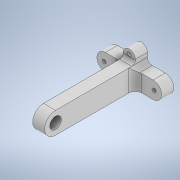
# Autodesk Inventor part: Motor Mount V2
Saved by Autodesk Inventor 2020 (Build 240168000, 168)
## iProperties
Created: 2022-04-04
Part Number: Motor Mount V2
Material: Generic
Document SubType Name: Modeling
Designer: maxwe
Density: 1 g/cm^3
Appearance: Default
Author: maxwe
Autodesk Inventor part; units mm, degrees
ref_plane "YZ Plane" through (0, 0, 0) normal (1, 0, 0) x (0, 1, 0)
ref_plane "XZ Plane" through (0, 0, 0) normal (0, 1, 0) x (-1, 0, 0)
ref_plane "XY Plane" through (0, 0, 0) normal (0, 0, 1) x (1, 0, 0)
sketch "Sketch1" plane through (0, 0, 0) normal (1, 0, 0) x (0, 1, 0)
  line L0 (0, 0) -> (17.9, 0)
  line L1 (17.9, 0) -> (17.9, 85)
  line L2 (17.9, 85) -> (0, 85)
  line L3 (0, 85) -> (0, 0)
  dimension "d0" = 17.9
  dimension "d1" = 85
  constraints: 8 end point, 2 parallel, 1 horizontal, 1 perpendicular
  measures "d0" distance of L2.end L1.end
  measures "d1" distance of L1.end L0.end
extrude "Extrusion1" add sketch "Sketch1" along normal blind 10
fillet "Fillet1" radius 8.95 2 edges at (5, 17.9, 85) (5, 0, 85)
sketch "Sketch2" plane through (10, 0, 0) normal (1, 0, 0) x (0, 0, -1)
  arc A0 (-76.05, 17.9) -> (-76.05, 0) centre (-76.05, 8.95) ccw projected
  circle A1 centre (-76.05, 8.95) radius 4.75
  point P0 (0, 0)
  dimension "d5" = 9.5
  constraints: 1 centre point, 1 coincident
  measures "d5" diameter of A1
extrude "Extrusion2" cut sketch "Sketch2" against normal blind 10
sketch "Sketch3" plane through (0, 0, 0) normal (0, 0, -1) x (-1, 0, 0)
  line L0 (14.8, 0) -> (-24.8, 0)
  line L1 (-31.8, 7) -> (-31.8, 7)
  line L2 (-24.8, 14) -> (14.8, 14)
  line L3 (21.8, 7) -> (21.8, 7)
  line L4 (0, 0) -> (0, 17.9) projected
  line L5 (-10, 0) -> (-10, 17.9) projected
  line L6 (0, 17.9) -> (-10, 17.9) projected
  circle A0 centre (-25.7, 7) radius 1.6
  circle A1 centre (15.7, 7) radius 1.6
  arc A2 (-24.8, 14) -> (-31.8, 7) centre (-24.8, 7) ccw
  arc A3 (-31.8, 7) -> (-24.8, 0) centre (-24.8, 7) ccw
  arc A4 (21.8, 7) -> (14.8, 14) centre (14.8, 7) ccw
  arc A5 (14.8, 0) -> (21.8, 7) centre (14.8, 7) ccw
  point P0 (21.8, 0)
  point P1 (-31.8, 14)
  point P2 (-31.8, 0)
  point P3 (21.8, 14)
  point P4 (-10, 14)
  point P5 (0, 14)
  point P6 (21.8, 7)
  point P7 (-31.8, 7)
  dimension "d8" = 14
  dimension "d9" = 21.8
  dimension "d10" = 21.8
  dimension "d11" = 17.9
  dimension "d12" = 3.2
  dimension "d13" = 3.2
  dimension "d14" = 6.1
  dimension "d15" = 6.1
  dimension "d16" = 7
  dimension "d17" = 7
  dimension "d23" = 7
  constraints: 8 end point, 8 point on circle, 8 point on line, 8 tangent, 6 centre point, 3 equal radius, 2 parallel, 1 horizontal, 1 perpendicular
  measures "d8" distance of point (21.8, 14) point (21.8, 0)
  measures "d9" distance between parallel lines of L4 L3
  measures "d10" distance between parallel lines of L5 L1
  measures "d11" distance between parallel lines of L6 L0
  measures "d12" diameter of A0
  measures "d13" diameter of A1
  measures "d14" distance from line of L1 A0.centre
  measures "d15" distance from line of L3 A1.centre
  measures "d16" distance from line of L2 A0.centre
  measures "d17" distance from line of L2 A1.centre
  measures "d23" radius of A2
extrude "Extrusion3" add sketch "Sketch3" against normal blind 10 contours L0 L4 L2 A4 A5 | L0 L5 L2 L4 | L0 A3 A2 L2 L5
fillet "Fillet3" radius 5.5 2 edges at (10, 7, 10) (0, 7, 10)
fillet "Fillet4" radius 3.9 4 edges at (0, 14, 12.75) (0, 14, 5) (10, 14, 12.75) (10, 14, 5)
sketch "Sketch4" plane through (24.8, 7, 0) normal (0, 0, -1) x (-1, 0, 0)
  line L0 (14.8, 10.9) -> (14.8, -7) projected
  line L1 (14.8, 10.9) -> (24.8, 10.9)
  line L2 (24.8, 10.9) -> (24.8, 14.4)
  line L3 (19.8, 19.4) -> (19.8, 19.4)
  line L4 (14.8, 14.4) -> (14.8, 10.9)
  circle A0 centre (19.8, 15.7) radius 1.6
  arc A1 (19.8, 19.4) -> (14.8, 14.4) centre (19.8, 14.4) ccw
  arc A2 (24.8, 14.4) -> (19.8, 19.4) centre (19.8, 14.4) ccw
  point P0 (24.8, -7)
  point P1 (24.8, 19.4)
  point P2 (19.8, 19.4)
  dimension "d24" = 8.5
  dimension "d25" = 3.2
  dimension "d26" = 4.8
  dimension "d27" = 5
  constraints: 8 end point, 4 point on circle, 4 tangent, 3 centre point, 2 parallel, 2 point on line, 1 concentric, 1 horizontal, 1 perpendicular
  measures "d24" distance of point (24.8, 19.4) L1.end
  measures "d25" diameter of A0
  measures "d26" distance from line of L1 A0.centre
  measures "d27" radius of A1
extrude "Extrusion4" add sketch "Sketch4" against normal blind 10
fillet "Fillet5" radius 3 1 edges at (5, 17.9, 10)
body "Solid1"
